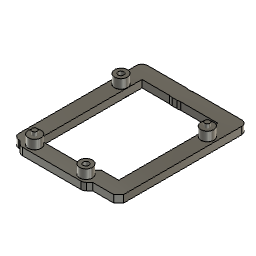
SpresenseExtensionBoardMount (Autodesk Fusion 360 design; units mm, degrees)
Autodesk Fusion 360 part; units mm, degrees
sketch "Sketch1" plane through (0, 0, 0) normal (0, 0, 1) x (1, 0, 0)
  arc A0 (38.1389, 0.2929) -> (37.4318, 0) centre (37.4318, 1) cw
  line L0 (53.34, 67.58) -> (53.34, 4.064)
  arc A1 (22.447, 68.58) -> (22.88, 68.33) centre (22.88, 68.83) ccw
  line L1 (25.813, 68.58) -> (52.34, 68.58)
  line L2 (1, 68.58) -> (22.447, 68.58)
  line L3 (0, 3.54) -> (0, 67.58)
  arc A2 (5.4942, 0) -> (4.7871, 0.2929) centre (5.4942, 1) cw
  line L4 (40.386, 2.54) -> (38.1389, 0.2929)
  line L5 (4.7871, 0.2929) -> (2.54, 2.54)
  line L6 (22.88, 68.33) -> (25.38, 68.33)
  line L7 (37.4318, 0) -> (5.4942, 0)
  line L8 (2.54, 2.54) -> (1, 2.54)
  arc A3 (52.34, 68.58) -> (53.34, 67.58) centre (52.34, 67.58) cw
  line L9 (51.816, 2.54) -> (40.386, 2.54)
  arc A4 (0, 67.58) -> (1, 68.58) centre (1, 67.58) cw
  arc A5 (25.38, 68.33) -> (25.813, 68.58) centre (25.38, 68.83) ccw
  line L10 (53.34, 4.064) -> (51.816, 2.54)
  arc A6 (1, 2.54) -> (0, 3.54) centre (1, 3.54) cw
  circle A7 centre (2.54, 54.61) radius 1.55
  circle A8 centre (50.8, 53.34) radius 1.4
  circle A9 centre (35.56, 2.54) radius 1.55
  circle A10 centre (7.62, 2.54) radius 1.4
  line L11 (23.4152, 70.33) -> (24.8448, 70.33)
  arc A11 (25.813, 70.58) -> (24.8448, 70.33) centre (25.813, 68.58) ccw
  line L12 (25.813, 70.58) -> (52.34, 70.58)
  arc A12 (55.34, 67.58) -> (52.34, 70.58) centre (52.34, 67.58) ccw
  line L13 (55.34, 67.58) -> (55.34, 3.2356)
  line L14 (55.34, 3.2356) -> (52.6444, 0.54)
  line L15 (52.6444, 0.54) -> (41.2144, 0.54)
  line L16 (41.2144, 0.54) -> (39.5531, -1.1213)
  arc A13 (37.4318, -2) -> (39.5531, -1.1213) centre (37.4318, 1) ccw
  line L17 (37.4318, -2) -> (5.4942, -2)
  arc A14 (3.3729, -1.1213) -> (5.4942, -2) centre (5.4942, 1) ccw
  line L18 (3.3729, -1.1213) -> (1.7116, 0.54)
  line L19 (1.7116, 0.54) -> (1, 0.54)
  arc A15 (-2, 3.54) -> (1, 0.54) centre (1, 3.54) ccw
  line L20 (-2, 3.54) -> (-2, 67.58)
  arc A16 (1, 70.58) -> (-2, 67.58) centre (1, 67.58) ccw
  line L21 (1, 70.58) -> (22.447, 70.58)
  arc A17 (23.4152, 70.33) -> (22.447, 70.58) centre (22.447, 68.58) ccw
  circle A18 centre (50.8, 53.34) radius 3.5
  circle A19 centre (35.56, 2.54) radius 3.5
  circle A20 centre (7.62, 2.54) radius 3.5
  circle A21 centre (2.54, 54.61) radius 3.5
  line L22 (47.2351, 62.4751) -> (47.2351, 8.6449)
  line L23 (47.2351, 8.6449) -> (37.8573, 8.6449)
  line L24 (37.8573, 8.6449) -> (35.3173, 6.1049)
  line L25 (35.3173, 6.1049) -> (7.6087, 6.1049)
  line L26 (7.6087, 6.1049) -> (6.1049, 7.6087)
  line L27 (6.1049, 7.6087) -> (6.1049, 62.4751)
  line L28 (6.1049, 62.4751) -> (21.08, 62.4751)
  arc A22 (21.08, 62.4751) -> (22.88, 62.2251) centre (22.88, 68.83) ccw
  line L29 (22.88, 62.2251) -> (25.38, 62.2251)
  arc A23 (25.38, 62.2251) -> (27.18, 62.4751) centre (25.38, 68.83) ccw
  line L30 (27.18, 62.4751) -> (47.2351, 62.4751)
  dimension "d1" = 3.1
  dimension "d2" = 2.8
  dimension "d3" = 2.8
  dimension "d8" = -2
  dimension "d9" = 7
  dimension "d10" = 7
  dimension "d11" = 3.1
  dimension "d12" = 7
  dimension "d13" = 7
  dimension "d14" = 6.1049
  constraint concentric A8 A18
  constraint concentric A9 A19
  constraint concentric A10 A20
  constraint concentric A7 A21
  measures "d1" diameter of A9
  measures "d2" diameter of A10
  measures "d3" diameter of A8
  measures "d9" diameter of A21
  measures "d10" diameter of A20
  measures "d11" diameter of A7
  measures "d12" diameter of A19
  measures "d13" diameter of A18
extrude "Extrude2" add sketch "Sketch1" along normal blind 5 contours A0 L4 L7 A19 | A0 L4 L7 A19 | A2 L7 A20 | A2 L7 A20 | L0 A18 | L0 A18 | L3 A21 | L3 A21 | A7 | A8 | A9 | A10 makes body 1 at (11.1026, 2.1915, 1.6667) makes body 2 at (6.0226, 54.2615, 1.6667) makes body 3 at (39.0426, 2.8885, 3.3333) makes body 4 at (54.2826, 53.6885, 3.3333)
extrude "Extrude3" add sketch "Sketch1" along normal blind 7 separate body contours A8 | A10 makes body 5 at (49.6054, 52.61, 4.6667) makes body 6 at (9.0183, 2.4702, 4.6667)
extrude "Extrude4" add sketch "Sketch1" against normal blind 4 separate body contours L0 A1 L1 L2 L3 A2 L4 L5 L6 L7 L8 A3 L9 A4 A5 L10 A6 A18 A19 A20 A21 | L11 A11 L12 A12 L13 L14 L15 L16 A13 L17 A14 L18 L19 A15 L20 A16 L21 A17 makes body 7
sketch "Sketch2" plane through (0, 0, 5) normal (0, 0, 1) x (-1, 0, 0)
  circle A0 centre (-2.54, -54.61) radius 3.5
  circle A1 centre (-2.54, -54.61) radius 1.55
  dimension "d21" = 3.1
  constraint concentric A0 A1
  measures "d21" diameter of A1
extrude "Extrude5" cut sketch "Sketch2" against normal blind 5 contours A1 bodies 2
sketch "Sketch3" plane through (0, 0, 5) normal (0, 0, 1) x (-1, 0, 0)
  circle A0 centre (-35.56, -2.54) radius 3.5
  circle A1 centre (-35.56, -2.54) radius 1.55
  dimension "d24" = 3.1
  constraint concentric A0 A1
  measures "d24" diameter of A1
extrude "Extrude6" cut sketch "Sketch3" against normal blind 5 contours A1 bodies 3
extrude "Extrude7" add sketch "Sketch1" against normal up to surface (4 mm away) separate body contours A0 L4 L7 A19 | A0 L4 L7 A19 | A2 L7 A20 | A2 L7 A20 | L0 A18 | L0 A18 | L3 A21 | L3 A21 | A7 | A8 | A9 | A10 makes body 8 at (11.1156, 2.3655, -2.6667) makes body 9 at (6.0356, 54.4355, -2.6667) makes body 10 at (39.0426, 2.8885, -1.3333) makes body 11 at (54.2826, 53.6885, -1.3333)
equation "d1 = d11"
equation "d2 = d3"
equation "MountHeight = 5 mm"
equation "d10 = d9"
equation "d12 = d9"
equation "d13 = d9"
equation "d15 = MountHeight"
equation "d17 = MountHeight + 2 mm"
